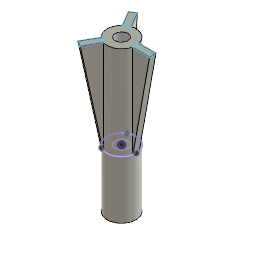
Kindergitter (Autodesk Fusion 360 design; units mm, degrees)
Autodesk Fusion 360 part; units mm, degrees
sketch "Sketch1" plane through (0, 0, 0) normal (0, 1, 0) x (1, 0, 0)
  circle A0 centre (0, 0) radius 1.95
  circle A1 centre (0, 0) radius 4.5
  dimension "d1" = 3.9
  dimension "d2" = 9
  constraint coincident A0.centre A1.centre
  constraint concentric A0 A1
  measures "d1" diameter of A0
  measures "d2" diameter of A1
extrude "Extrude1" add sketch "Sketch1" along normal blind 47
ref_plane "WorkPlane1" through (0, 18, 0) normal (0, 1, 0) x (0, 0, 1)
sketch "Sketch2" plane through (0, 18, 0) normal (0, 1, 0) x (1, 0, 0)
  circle A0 centre (0, 0) radius 4.5
  line L0 (4.5249, -1) -> (4.3, -1)
  line L1 (4.3, -1) -> (4.3, 1)
  line L2 (4.3, 1) -> (4.5249, 1)
  line L3 (4.5249, 1) -> (4.5249, -1)
  line L4 (4.5249, -1) -> (4.3, 1) construction
  line L5 (4.3, -1) -> (4.5249, 1) construction
  circle A1 centre (0, 0) radius 4.5
  circle A2 centre (0, 0) radius 1.95
  circle A3 centre (0, 0) radius 4.5
  line L6 (-1.284, 4.2239) -> (-3.016, 3.2239)
  line L7 (-3.016, 3.2239) -> (-3.1285, 3.4187)
  line L8 (-1.3964, 4.4187) -> (-1.284, 4.2239)
  line L9 (-3.1285, 3.4187) -> (-1.3964, 4.4187)
  line L10 (-1.3964, 4.4187) -> (-3.016, 3.2239) construction
  line L11 (-1.284, 4.2239) -> (-3.1285, 3.4187) construction
  line L12 (-3.1285, -3.4187) -> (-3.016, -3.2239)
  line L13 (-1.284, -4.2239) -> (-1.3964, -4.4187)
  line L14 (-3.1285, -3.4187) -> (-1.284, -4.2239) construction
  line L15 (-3.016, -3.2239) -> (-1.3964, -4.4187) construction
  line L16 (-1.3964, -4.4187) -> (-3.1285, -3.4187)
  line L17 (-3.016, -3.2239) -> (-1.284, -4.2239)
  point P0 (4.4125, 0)
  point P1 (-2.2062, 3.8213)
  point P2 (-2.2062, -3.8213)
  dimension "d6" = 9
  dimension "d7" = 2
  dimension "d13" = 2
  dimension "d14" = 2
  constraint coincident A0.centre A1.centre
  constraint horizontal L0
  constraint perpendicular L0 L1
  constraint parallel L0 L2
  constraint parallel L1 L3
  constraint coincident L4 P0
  constraint coincident L5 P0
  constraint perpendicular L6 L8
  constraint parallel L7 L8
  constraint parallel L6 L9
  constraint coincident P1 L10
  constraint coincident P1 L11
  constraint perpendicular L12 L17
  constraint parallel L12 L13
  constraint parallel L16 L17
  constraint coincident P2 L14
  constraint coincident P2 L15
  measures "d6" diameter of A0
  measures "d7" distance of L0.end L1.end
  measures "d13" distance of L6.end L6.start
  measures "d14" distance of L13.start L12.end
sketch "Sketch3" plane through (0, 47, 0) normal (0, 1, 0) x (-1, 0, 0)
  circle A0 centre (0, 0) radius 1.95
  circle A1 centre (0, 0) radius 4.5
  line L0 (-4.3, -1) -> (-9.7, -1)
  line L1 (-9.7, -1) -> (-9.7, 1)
  line L2 (-9.7, 1) -> (-4.3, 1)
  line L3 (-4.3, 1) -> (-4.3, -1)
  line L4 (3.984, -8.9004) -> (1.284, -4.2239)
  line L5 (3.016, -3.2239) -> (5.716, -7.9004)
  line L6 (5.716, -7.9004) -> (3.984, -8.9004)
  line L7 (1.284, -4.2239) -> (3.016, -3.2239)
  line L8 (3.984, 8.9004) -> (5.716, 7.9004)
  line L9 (3.016, 3.2239) -> (1.284, 4.2239)
  line L10 (5.716, 7.9004) -> (3.016, 3.2239)
  line L11 (1.284, 4.2239) -> (3.984, 8.9004)
  dimension "d10" = 5.4
  dimension "d11" = 5.4
  dimension "d12" = 5.4
  constraint horizontal L0
  constraint vertical L1
  constraint horizontal L2
  constraint vertical L3
  measures "d10" distance of L0.start L0.end
  measures "d11" distance of L5.start L5.end
  measures "d12" distance of L9.end L8.start
loft "Loft1" add profiles "Sketch2", "Sketch3" section 1 contours A0 L0 L2 L3 A1 A3 section 2 contours A1 L0 L1 L2
loft "Loft2" add profiles "Sketch2", "Sketch3" section 1 contours A0 A1 A3 L12 L13 L16 section 2 contours A1 L8 L10 L11
loft "Loft3" add profiles "Sketch2", "Sketch3" section 1 contours A0 A1 A3 L7 L8 L9 section 2 contours A1 L4 L5 L6
